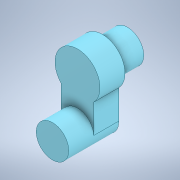
# Autodesk Inventor part: Component37
Saved by Autodesk Inventor 2022 (Build 260153000, 153)
## iProperties
Created: 2022-01-29
Part Number: Component37
Material: Generic
Document SubType Name: Modeling
Designer: Administrator
Density: 1 g/cm^3
Appearance: Default
Title: Component37
Author: Administrator
Autodesk Inventor part; units mm, degrees
ref_plane "YZ Plane" through (0, 0, 0) normal (1, 0, 0) x (0, 1, 0)
ref_plane "XZ Plane" through (0, 0, 0) normal (0, 1, 0) x (-1, 0, 0)
ref_plane "XY Plane" through (0, 0, 0) normal (0, 0, 1) x (1, 0, 0)
sketch "Sketch2" plane through (0, 0, 0) normal (0, 0, 1) x (1, 0, 0)
  arc A0 (3.248, -2.1196) -> (-3.248, -2.1196) centre (0, 0.995) ccw
  line L0 (-3.248, -7.8914) -> (-3.248, -2.1196)
  circle A1 centre (0, -8.005) radius 3.25
  circle A2 centre (0, 0.995) radius 3.25
  line L1 (0, -15.3117) -> (0, 6.7515) construction
  line L2 (3.248, -7.8914) -> (3.248, -2.1196)
  point P0 (0, 0)
  point P1 (-2.9785, -8.0287)
  dimension "d6" = 6.5
  dimension "d7" = 9
  dimension "d8" = 9
  constraints: 6 end point, 2 centre point, 2 point on circle, 2 point on line, 2 symmetric about line, 1 coincident, 1 parallel, 1 vertical, 4 other
  measures "d7" diameter of A0
  measures "d8" distance of point (0, -8.005) A0.centre
extrude "Extrusion1" add sketch "Sketch2" against normal blind 5 contours L2 A1 L0 A0 | A1 | A2
extrude "Extrusion2" add sketch "Sketch2" along normal blind 5 contours A1
sketch "Sketch3" plane through (0, 0, -5) normal (0, 0, -1) x (-1, 0, 0)
  circle A0 centre (0, 0.995) radius 3.25 projected
  point P0 (0, 0)
extrude "Extrusion3" add sketch "Sketch3" along normal blind 5
equation "\"d6\" = R"
equation "\"d7\" = R1"
equation "\"d0\" = thickness"
equation "\"d2\" = thickness"
equation "\"d4\" = thickness"
equation "\"R\" = 6.5"
equation "\"thickness\" = 5"
equation "\"width\" = 6.5"
equation "\"R1\" = 9"
body "Solid1"
